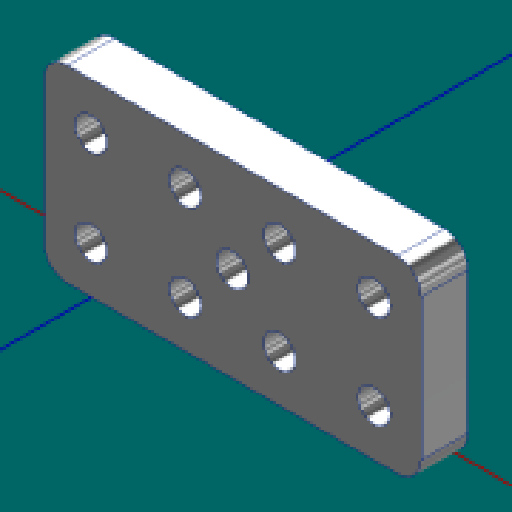
# Autodesk Inventor part: IntakeShoulder
Saved by Autodesk Inventor 2023.1 (Build 271208000, 208)
## iProperties
Created: 2022-11-06
Part Number: IntakeShoulder
Material: Aluminum 6061
Document SubType Name: Modeling
Designer: zac-h
Density: 2.7 g/cm^3
Appearance: Aluminum - Flat
Mass: 11.2632 g
Surface Area: 43.63 cm^2
Volume: 4.17154 cm^3
Author: zac-h
Autodesk Inventor part; units mm, degrees
ref_plane "YZ Plane" through (0, 0, 0) normal (1, 0, 0) x (0, 1, 0)
ref_plane "XZ Plane" through (0, 0, 0) normal (0, 1, 0) x (-1, 0, 0)
ref_plane "XY Plane" through (0, 0, 0) normal (0, 0, 1) x (1, 0, 0)
sketch "Sketch1" plane through (0, 0, 0) normal (0, 0, 1) x (1, 0, 0)
  circle A0 centre (0, 0) radius 2.159
  line L0 (0, 0) -> (38.1, 0) construction
  line L1 (0, 0) -> (0, 12.7) construction
  circle A1 centre (12.7, 0) radius 2.159
  circle A2 centre (25.4, 0) radius 2.159
  circle A3 centre (38.1, 0) radius 2.159
  circle A4 centre (0, 12.7) radius 2.159
  circle A5 centre (12.7, 12.7) radius 2.159
  circle A6 centre (25.4, 12.7) radius 2.159
  circle A7 centre (38.1, 12.7) radius 2.159
  circle A8 centre (19.05, 6.35) radius 2.159
  line L2 (12.7, 12.7) -> (25.4, 0) construction
  line L3 (-6.35, 19.05) -> (44.45, 19.05)
  line L4 (44.45, 19.05) -> (44.45, -6.35)
  line L5 (44.45, -6.35) -> (-6.35, -6.35)
  line L6 (-6.35, -6.35) -> (-6.35, 19.05)
  circle A9 centre (0, 12.7) radius 6.35 construction
  circle A10 centre (38.1, 0) radius 6.35 construction
  dimension "d0" = 4.318
  dimension "d1" = 38.1
  dimension "d9" = 12.7
  dimension "d12" = 12.7
  dimension "d15" = 12.7
  dimension "d18" = 4.318
  dimension "d19" = 25.4
  constraints: 14 end point, 11 centre point, 4 tangent, 3 coincident, 3 horizontal, 2 parallel, 2 vertical, 1 equal radius, 1 midpoint, 1 perpendicular, 14 other
  measures "d0" diameter of A0
  measures "d1" distance of L0.start L0.end
  measures "d9" distance of L0.start L1.end
  measures "d12" distance of L0.start A1.centre
  measures "d15" distance of L0.start A4.centre
  measures "d18" diameter of A8
  measures "d19" distance of L3.end L4.end
extrude "Extrusion1" add sketch "Sketch1" along normal blind 6.35
fillet "Fillet1" radius 3.175 4 edges at (44.45, 19.05, 3.175) (44.45, -6.35, 3.175) (-6.35, -6.35, 3.175) (-6.35, 19.05, 3.175)
sketch "Sketch3" plane through (0, 0, 0) normal (0, 0, -1) x (-1, 0, 0)
  arc A0 (6.35, 15.875) -> (3.175, 19.05) centre (3.175, 15.875) ccw projected
  line L0 (-41.275, 19.05) -> (3.175, 19.05) projected
  arc A1 (-41.275, 19.05) -> (-44.45, 15.875) centre (-41.275, 15.875) ccw projected
  line L1 (-44.45, -3.175) -> (-44.45, 15.875) projected
  arc A2 (-44.45, -3.175) -> (-41.275, -6.35) centre (-41.275, -3.175) ccw projected
  line L2 (3.175, -6.35) -> (-41.275, -6.35) projected
  arc A3 (3.175, -6.35) -> (6.35, -3.175) centre (3.175, -3.175) ccw projected
  line L3 (6.35, 15.875) -> (6.35, -3.175) projected
  circle A4 centre (-19.05, 6.35) radius 2.159 projected
  circle A5 centre (0, 0) radius 2.159 projected
  circle A6 centre (-12.7, 0) radius 2.159 projected
  circle A7 centre (-25.4, 0) radius 2.159 projected
  circle A8 centre (-38.1, 0) radius 2.159 projected
  circle A9 centre (0, 12.7) radius 2.159 projected
  circle A10 centre (-12.7, 12.7) radius 2.159 projected
  circle A11 centre (-25.4, 12.7) radius 2.159 projected
  circle A12 centre (-38.1, 12.7) radius 2.159 projected
  line L4 (-21.59, 6.35) -> (-16.51, 6.35) construction
  line L5 (-21.59, 1.778) -> (-16.51, 1.778)
  line L6 (-16.51, 10.922) -> (-21.59, 10.922)
  arc A13 (-21.59, 10.922) -> (-21.59, 1.778) centre (-21.59, 6.35) ccw
  arc A14 (-16.51, 1.778) -> (-16.51, 10.922) centre (-16.51, 6.35) ccw
  dimension "d40" = 9.144
  dimension "d41" = 5.08
  constraints: 8 end point, 4 point on circle, 4 tangent, 2 centre point, 1 coincident, 1 horizontal, 1 midpoint, 1 parallel
  measures "d40" diameter of A14
  measures "d41" distance of L4.start L4.end
extrude "Extrusion3" cut sketch "Sketch3" against normal blind 1.5875 contours A4 | A13 L6 A14 L5
body "Solid1"
